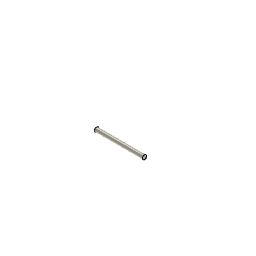
Long bolt Between Wheel and Gear (Autodesk Fusion 360 design; units mm, degrees)
Autodesk Fusion 360 part; units mm, degrees
sketch "Hole" plane through (70, 0, 0) normal (1, 0, 0) x (0, 1, 0)
  circle A0 centre (19.7806, 16.0772) radius 1.75
  dimension "d293" = 3.5
  measures "d293" diameter of A0
extrude "Extrude1" add sketch "Hole" along normal blind 12 and the other way blind 28
named bodies: "Middle Tube"
